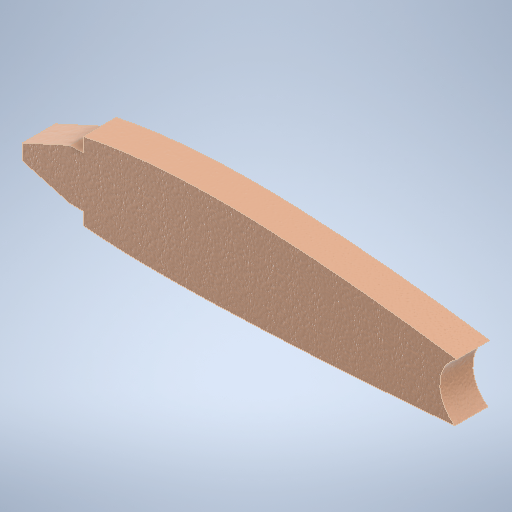
# Autodesk Inventor part: 2414 basic aerofoil
Saved by Autodesk Inventor 2025.2 (Build 292293000, 293)
## iProperties
Created: 2024-11-04
Part Number: 2414 basic aerofoil
Material: Polyurethane Foam
Document SubType Name: Modeling
Designer: johan
Density: 0.032 g/cm^3
Appearance: Coarse Textured - Umber
Author: johan
Autodesk Inventor part; units mm, degrees
ref_plane "YZ Plane" through (0, 0, 0) normal (1, 0, 0) x (0, 1, 0)
ref_plane "XZ Plane" through (0, 0, 0) normal (0, 1, 0) x (-1, 0, 0)
ref_plane "XY Plane" through (0, 0, 0) normal (0, 0, 1) x (1, 0, 0)
sketch "Sketch2" plane through (0, 0, 0) normal (0, 0, 1) x (1, 0, 0)
  spline S0 degree 5 poles (319.6498, 0.0573) (319.6501, 0.0612) (319.6024, 0.0717) (319.3745, 0.1032) (319.3587, 0.1577) (318.7204, 0.2502) (318.4411, 0.3675) (317.6227, 0.5236) (316.9347, 0.7102) (315.9239, 0.9334) (314.8763, 1.1861) (313.6258, 1.4728) (312.2675, 1.7887) (310.7514, 2.1347) (309.1071, 2.5099) (307.3204, 2.9131) (305.4017, 3.3421) (303.3481, 3.7974) (301.1639, 4.2757) (298.8502, 4.7782) (296.4092, 5.301) (293.8432, 5.8446) (291.1548, 6.4061) (288.3466, 6.9857) (285.4207, 7.5803) (282.3807, 8.1894) (279.2284, 8.8107) (275.968, 9.4437) (272.6016, 10.0865) (269.1329, 10.7361) (265.5656, 11.3942) (261.9019, 12.0551) (258.1469, 12.7207) (254.3029, 13.3883) (250.3742, 14.0555) (246.3647, 14.7217) (242.2776, 15.3854) (238.118, 16.0441) (233.8887, 16.6979) (229.5952, 17.3434) (225.2402, 17.981) (220.8297, 18.6074) (216.3658, 19.2226) (211.8552, 19.8242) (207.3009, 20.4107) (202.7077, 20.9813) (198.0804, 21.5339) (193.4232, 22.0679) (188.7413, 22.58) (184.0389, 23.0713) (179.321, 23.5382) (174.592, 23.982) (169.8567, 24.3971) (165.1201, 24.7874) (160.3872, 25.1472) (155.6604, 25.4776) (150.948, 25.7772) (146.2454, 26.0449) (141.5744, 26.278) (136.9015, 26.4795) (132.2479, 26.6311) (127.6319, 26.7393) (123.054, 26.7999) (118.5202, 26.8147) (114.0397, 26.7815) (109.6094, 26.7031) (105.2517, 26.5723) (100.9331, 26.4088) (96.7495, 26.1663) (92.5147, 25.9483) (88.6376, 25.5343) (84.2302, 25.3974) (81.2071, 24.5612) (76.5297, 24.5259) (73.18, 23.8676) (69.3619, 23.413) (65.9721, 22.8018) (62.3454, 22.244) (59.4319, 21.514) (55.4307, 21.0148) (53.2464, 20.1084) (49.5889, 19.537) (47.2944, 18.6473) (44.3884, 17.909) (41.914, 17.071) (39.4431, 16.2394) (37.1538, 15.3738) (34.9769, 14.4941) (32.9455, 13.5944) (31.0501, 12.6807) (29.2961, 11.7542) (27.6837, 10.8151) (26.2149, 9.8673) (24.8895, 8.9103) (23.7099, 7.9467) (22.6751, 6.976) (21.7868, 6.0004) (21.0458, 5.0186) (20.4526, 4.032) (20.0117, 3.0392) (19.7221, 2.0438) (19.5893, 1.0479) (19.6118, 0.0538) (19.7865, -0.9258) (20.1138, -1.8742) (20.591, -2.7944) (21.2165, -3.6796) (21.9855, -4.5321) (22.8956, -5.3514) (23.9453, -6.1385) (25.1332, -6.8944) (26.4582, -7.6188) (27.9184, -8.3123) (29.5136, -8.9751) (31.2409, -9.6071) (33.0997, -10.2067) (35.0892, -10.7758) (37.2002, -11.3131) (39.4562, -11.8174) (41.7927, -12.2939) (44.3651, -12.7275) (46.7744, -13.1584) (50.0005, -13.481) (52.1533, -13.8927) (55.9371, -14.1294) (58.2153, -14.4717) (61.732, -14.6854) (64.8012, -14.9153) (68.2287, -15.092) (71.6338, -15.2498) (75.1915, -15.3722) (78.8138, -15.4692) (82.5326, -15.5359) (86.3291, -15.5764) (90.2061, -15.5901) (94.1575, -15.5787) (98.1812, -15.5438) (102.2727, -15.4851) (106.4286, -15.4059) (110.6456, -15.3062) (114.9188, -15.1867) (119.2459, -15.0512) (123.6218, -14.8988) (128.0442, -14.7319) (132.5111, -14.552) (137.0141, -14.3592) (141.5621, -14.1606) (146.1675, -13.9403) (150.787, -13.7052) (155.434, -13.4523) (160.0951, -13.1857) (164.7676, -12.9046) (169.4465, -12.6129) (174.1261, -12.3082) (178.8033, -11.9955) (183.4722, -11.6727) (188.1294, -11.3426) (192.7696, -11.0072) (197.3886, -10.6641) (201.9818, -10.3188) (206.5448, -9.9678) (211.0728, -9.6157) (215.5623, -9.2611) (220.0069, -8.9047) (224.4048, -8.5497) (228.7492, -8.193) (233.0373, -7.8393) (237.2647, -7.4865) (241.4259, -7.1353) (245.5189, -6.7884) (249.5374, -6.4441) (253.4791, -6.104) (257.3389, -5.7683) (261.1136, -5.4376) (264.7987, -5.113) (268.3914, -4.7937) (271.8871, -4.4807) (275.2826, -4.1749) (278.5752, -3.8759) (281.7596, -3.585) (284.8354, -3.3021) (287.7962, -3.0278) (290.6419, -2.763) (293.3672, -2.5063) (295.9712, -2.2616) (298.4496, -2.0246) (300.8012, -1.801) (303.0222, -1.5859) (305.1122, -1.3849) (307.0656, -1.194) (308.8864, -1.0166) (310.5623, -0.8504) (312.1091, -0.6993) (313.4945, -0.5587) (314.7717, -0.4371) (315.8415, -0.3205) (316.8737, -0.2329) (317.5782, -0.1363) (318.4119, -0.0906) (318.7016, -0.0103) (319.3493, -0.0034) (319.3699, 0.0485) (319.6005, 0.0494) (319.6495, 0.0534) (319.6498, 0.0573) knots 0 0 0 0 0 0 0.001406 0.002637 0.004353 0.006443 0.008834 0.011487 0.014375 0.017478 0.020781 0.02427 0.027934 0.031762 0.035746 0.039878 0.044151 0.048559 0.053094 0.057751 0.062526 0.067412 0.072404 0.077499 0.082692 0.087977 0.093351 0.098811 0.104351 0.109968 0.115658 0.121418 0.127243 0.133131 0.139077 0.145079 0.151132 0.157233 0.163379 0.169567 0.175793 0.182054 0.188346 0.194667 0.201013 0.20738 0.213767 0.220168 0.226582 0.233004 0.239433 0.245864 0.252294 0.258721 0.265141 0.27155 0.27795 0.284339 0.290715 0.297074 0.303413 0.309725 0.316005 0.32225 0.328456 0.33462 0.340739 0.34681 0.352829 0.358735 0.364639 0.370482 0.376261 0.381971 0.38767 0.393236 0.398773 0.404177 0.409526 0.414755 0.419891 0.424884 0.429828 0.434638 0.439375 0.444 0.448512 0.452907 0.457182 0.461332 0.465356 0.469251 0.473017 0.476652 0.480158 0.48354 0.486805 0.489964 0.493033 0.496034 0.498989 0.501921 0.504852 0.507807 0.510807 0.513873 0.517028 0.520286 0.523658 0.527152 0.530771 0.534516 0.538388 0.542384 0.546503 0.550741 0.555095 0.559563 0.56414 0.568856 0.57364 0.578576 0.583553 0.588622 0.593747 0.598989 0.604262 0.609667 0.615146 0.620698 0.626318 0.632003 0.637751 0.643558 0.649421 0.655338 0.661304 0.667318 0.673375 0.679474 0.685611 0.691783 0.697987 0.704223 0.710491 0.716788 0.723111 0.729457 0.73582 0.742195 0.748576 0.754963 0.761351 0.767737 0.774118 0.780492 0.786854 0.793202 0.799533 0.805843 0.812129 0.818388 0.824617 0.830812 0.836971 0.843089 0.849164 0.855191 0.861169 0.867092 0.872959 0.878764 0.884505 0.890178 0.895778 0.901303 0.906749 0.91211 0.917384 0.922566 0.927651 0.932635 0.937513 0.942281 0.946932 0.951462 0.955865 0.960134 0.964263 0.968244 0.97207 0.975732 0.979219 0.982521 0.985624 0.988511 0.991164 0.993554 0.995643 0.997359 0.998591 1 1 1 1 1 1
  line L0 (79.5135, 4.6359) -> (79.5135, 24.6083) construction
  line L1 (79.5135, 4.6359) -> (209.6498, 4.6359) construction
  line L2 (319.6498, 0.0573) -> (219.6498, 0.0573) construction
  line L3 (219.6499, 18.7671) -> (219.6499, -8.9327) construction
  line L4 (28.0055, 4.5054) -> (28.0055, -2.4946)
  line L5 (19.627, 1.0326) -> (319.6498, 0.0573) construction
  line L6 (49.7105, 14.4213) -> (55.6079, 14.4213)
  line L7 (49.7104, -8.4915) -> (55.6078, -8.4915)
  line L8 (28.0055, 4.5054) -> (49.7105, 14.4213)
  line L9 (28.0055, -2.4946) -> (49.7104, -8.4915)
  line L10 (55.6079, 14.4213) -> (55.6079, 20.8726)
  line L11 (55.6078, -8.4915) -> (55.6078, -14.1513)
  arc A0 (225.2869, 17.9694) -> (224.4503, -8.5446) centre (233.3969, 4.4433) ccw
  point P0 (0, 0)
  point P1 (319.3573, 0.1272)
  point P2 (318.9918, 0.2142)
  point P3 (318.4802, 0.3354)
  point P4 (317.8238, 0.4911)
  point P5 (317.0222, 0.6801)
  point P6 (316.0769, 0.9024)
  point P7 (314.9885, 1.1568)
  point P8 (313.7582, 1.443)
  point P9 (312.3866, 1.7598)
  point P10 (310.8752, 2.1063)
  point P11 (309.2258, 2.4819)
  point P12 (307.4393, 2.8854)
  point P13 (305.5178, 3.3153)
  point P14 (303.4628, 3.7707)
  point P15 (301.2764, 4.2501)
  point P16 (298.9607, 4.7526)
  point P17 (296.5175, 5.2764)
  point P18 (293.9492, 5.8203)
  point P19 (291.2585, 6.3828)
  point P20 (288.4478, 6.9627)
  point P21 (285.5195, 7.5582)
  point P22 (282.4766, 8.1678)
  point P23 (279.3218, 8.79)
  point P24 (276.0584, 9.4236)
  point P25 (272.6891, 10.0668)
  point P26 (269.2175, 10.7178)
  point P27 (265.6469, 11.3757)
  point P28 (261.9803, 12.0381)
  point P29 (258.2219, 12.7041)
  point P30 (254.3747, 13.3722)
  point P31 (250.4426, 14.0403)
  point P32 (246.4295, 14.7072)
  point P33 (242.339, 15.3714)
  point P34 (238.1756, 16.0311)
  point P35 (233.9428, 16.6851)
  point P36 (229.6454, 17.3316)
  point P37 (220.8723, 18.5967)
  point P38 (216.4049, 19.2123)
  point P39 (211.8901, 19.8144)
  point P40 (207.332, 20.4015)
  point P41 (202.7347, 20.9724)
  point P42 (198.1034, 21.5256)
  point P43 (193.4423, 22.0596)
  point P44 (188.7563, 22.5726)
  point P45 (184.0499, 23.0637)
  point P46 (179.3279, 23.5314)
  point P47 (174.5948, 23.9745)
  point P48 (169.8554, 24.3909)
  point P49 (165.1148, 24.7803)
  point P50 (160.3775, 25.1406)
  point P51 (155.6479, 25.4709)
  point P52 (150.9316, 25.7703)
  point P53 (146.233, 26.0373)
  point P54 (141.557, 26.2707)
  point P55 (136.882, 26.4681)
  point P56 (132.2209, 26.6211)
  point P57 (127.5964, 26.7282)
  point P58 (123.0133, 26.7888)
  point P59 (118.4761, 26.8026)
  point P60 (113.9902, 26.7693)
  point P61 (109.5601, 26.6886)
  point P62 (105.191, 26.5611)
  point P63 (100.8866, 26.3866)
  point P64 (96.6524, 26.1647)
  point P65 (92.4927, 25.8975)
  point P66 (88.4121, 25.5832)
  point P67 (84.4152, 25.2282)
  point P68 (80.9052, 24.7441)
  point P69 (76.6873, 24.3761)
  point P70 (72.9635, 23.8905)
  point P71 (69.3402, 23.3611)
  point P72 (65.8208, 22.7938)
  point P73 (62.4086, 22.1883)
  point P74 (59.107, 21.5464)
  point P75 (52.8493, 20.1606)
  point P76 (49.7105, 19.4213)
  point P77 (47.0737, 18.6507)
  point P78 (44.3741, 17.8542)
  point P79 (41.8034, 17.0322)
  point P80 (39.3638, 16.1874)
  point P81 (37.0583, 15.3213)
  point P82 (34.8884, 14.4363)
  point P83 (32.8568, 13.534)
  point P84 (30.965, 12.6166)
  point P85 (29.2145, 11.686)
  point P86 (27.6071, 10.7437)
  point P87 (26.1443, 9.7921)
  point P88 (24.8269, 8.8324)
  point P89 (23.6566, 7.8664)
  point P90 (22.6336, 6.8953)
  point P91 (21.7591, 5.9209)
  point P92 (21.0334, 4.9441)
  point P93 (20.4571, 3.9661)
  point P94 (20.0308, 2.9875)
  point P95 (19.7539, 2.0098)
  point P96 (19.6496, 0.0573)
  point P97 (19.8205, -0.9033)
  point P98 (20.1376, -1.8357)
  point P99 (20.6002, -2.7402)
  point P100 (21.208, -3.6159)
  point P101 (21.9598, -4.4628)
  point P102 (22.8544, -5.2806)
  point P103 (23.8909, -6.069)
  point P104 (25.0681, -6.8277)
  point P105 (26.3846, -7.5561)
  point P106 (27.8384, -8.2539)
  point P107 (29.4284, -8.9211)
  point P108 (31.1522, -9.5571)
  point P109 (33.0086, -10.1613)
  point P110 (34.9949, -10.734)
  point P111 (37.1093, -11.2746)
  point P112 (39.3497, -11.7828)
  point P113 (41.7134, -12.2586)
  point P114 (44.198, -12.702)
  point P115 (46.8014, -13.1127)
  point P116 (49.7104, -13.4915)
  point P117 (52.3532, -13.8357)
  point P118 (58.3469, -14.4294)
  point P119 (61.5023, -14.6781)
  point P120 (64.7591, -14.8953)
  point P121 (68.1149, -15.0813)
  point P122 (71.5661, -15.237)
  point P123 (75.1094, -15.3627)
  point P124 (78.7418, -15.4596)
  point P125 (82.46, -15.528)
  point P126 (86.2607, -15.5691)
  point P127 (90.14, -15.5838)
  point P128 (94.0946, -15.5733)
  point P129 (98.1212, -15.5388)
  point P130 (102.2159, -15.4812)
  point P131 (106.3751, -15.4023)
  point P132 (110.5952, -15.303)
  point P133 (114.872, -15.1845)
  point P134 (119.2022, -15.0489)
  point P135 (123.5813, -14.8971)
  point P136 (128.006, -14.7306)
  point P137 (132.4718, -14.5509)
  point P138 (136.9748, -14.3598)
  point P139 (141.5285, -14.1576)
  point P140 (146.1365, -13.9383)
  point P141 (150.7679, -13.7022)
  point P142 (155.4191, -13.4499)
  point P143 (160.0853, -13.1829)
  point P144 (164.7617, -12.9024)
  point P145 (169.4444, -12.6099)
  point P146 (174.1283, -12.306)
  point P147 (178.8092, -11.9925)
  point P148 (183.4823, -11.67)
  point P149 (188.1434, -11.34)
  point P150 (192.7877, -11.0037)
  point P151 (197.4106, -10.6614)
  point P152 (202.0079, -10.3149)
  point P153 (206.5747, -9.9645)
  point P154 (211.1069, -9.6117)
  point P155 (215.5999, -9.2568)
  point P156 (220.0489, -8.9007)
  point P157 (228.7987, -8.1885)
  point P158 (233.0906, -7.8339)
  point P159 (237.3214, -7.4808)
  point P160 (241.4866, -7.1298)
  point P161 (245.5828, -6.7821)
  point P162 (249.6052, -6.4377)
  point P163 (253.5502, -6.0972)
  point P164 (257.4136, -5.7612)
  point P165 (261.1915, -5.4303)
  point P166 (264.88, -5.1051)
  point P167 (268.4758, -4.7856)
  point P168 (271.9747, -4.4724)
  point P169 (275.3734, -4.1661)
  point P170 (278.6686, -3.867)
  point P171 (281.8564, -3.5757)
  point P172 (284.9344, -3.2925)
  point P173 (287.8984, -3.018)
  point P174 (290.7463, -2.7525)
  point P175 (293.4745, -2.4963)
  point P176 (296.0806, -2.2503)
  point P177 (298.5616, -2.0142)
  point P178 (300.9151, -1.7892)
  point P179 (303.1387, -1.575)
  point P180 (305.23, -1.3728)
  point P181 (307.1866, -1.1823)
  point P182 (309.007, -1.0041)
  point P183 (310.6885, -0.8385)
  point P184 (312.2302, -0.6861)
  point P185 (313.6297, -0.5472)
  point P186 (314.8861, -0.4221)
  point P187 (315.9976, -0.3108)
  point P188 (316.9636, -0.2139)
  point P189 (317.7826, -0.1314)
  point P190 (318.4537, -0.0636)
  point P191 (318.9766, -0.0108)
  point P192 (319.3503, 0.027)
  point P193 (319.5743, 0.0498)
  point P194 (209.6498, 0.0573)
  point P195 (28.0055, 1.0054)
  point P196 (217.627, 4.6359)
  dimension "d2" = 300.0001
  dimension "d19" = 110
  dimension "d22" = 100
  dimension "d23" = 7
  dimension "d24" = 5
  dimension "d25" = 5
  dimension "d44" = 198
  dimension "d46" = 59.8865
  constraints: 24 end point, 4 vertical, 3 point on circle, 2 horizontal, 1 centre point, 1 horizontal alignment, 1 midpoint, 1 parallel, 1 point on line, 203 other
  measures "d2" distance of L2.start point (19.65, 0.057)
  measures "d19" distance of L2.start point (209.65, 0.057)
  measures "d22" distance of L2.start L2.end
  measures "d23" distance of L4.start L4.end
  measures "d24" distance from line of point (49.71, 19.421) L6
  measures "d25" distance from line of point (49.71, -13.491) L7
  measures "d44" horizontal distance of L5.start point (217.627, 4.636)
  measures "d46" horizontal distance of L5.start L0.start
extrude "Extrusion6" add sketch "Sketch2" along normal blind 15 contours A0 S0 L11 L7 L9 L4 L8 L6 L10
body "Solid6"
